Bielle sup (Autodesk Fusion 360 design; units mm, degrees)
Autodesk Fusion 360 part; units mm, degrees
sketch "Sketch1" plane through (0, 0, 0) normal (0, 0, 1) x (1, 0, 0) in component "Grande Bielle"
  line L0 (-178.5, 0) -> (178.5, 0) construction
  line L1 (-20, -20) -> (20, -20)
  line L2 (-32.5, 20) -> (-165, 7.5464)
  line L3 (20, -20) -> (165, -7.4425)
  line L4 (-20, -20) -> (-165, -7.4425)
  circle A0 centre (-178.5, 0) radius 3 construction
  line L5 (32.5, 20) -> (165, 7.5464)
  line L6 (0, 20) -> (0, -20) construction
  circle A1 centre (178.5, 0) radius 3 construction
  line L7 (32.5, 20) -> (32.5, 25)
  line L8 (32.5, 25) -> (-32.5, 25)
  line L9 (-32.5, 25) -> (-32.5, 20)
  line L10 (19.4422, 5.1) -> (-19.4422, -5.1) construction
  line L11 (-19.4422, 5.1) -> (19.4422, -5.1) construction
  arc A2 (-19.4422, 5.1) -> (-19.4422, -5.1) centre (0, 0) ccw
  arc A3 (19.4422, -5.1) -> (19.4422, 5.1) centre (0, 0) ccw
  line L12 (-32.5, 20) -> (32.5, 20) construction
  arc A4 (-14.2127, -5.1) -> (14.2127, -5.1) centre (0, 0) ccw
  arc A5 (14.2127, 5.1) -> (-14.2127, 5.1) centre (0, 0) ccw
  line L13 (19.4422, 5.1) -> (14.2127, 5.1)
  line L14 (-14.2127, 5.1) -> (-19.4422, 5.1)
  line L15 (-19.4422, -5.1) -> (-14.2127, -5.1)
  line L16 (14.2127, -5.1) -> (19.4422, -5.1)
  line L17 (-165, 7.5464) -> (-165, -7.4425)
  circle A6 centre (-155, 0) radius 2.1
  circle A7 centre (-145, 0) radius 2.1
  line L18 (165, 7.5464) -> (165, -7.4425)
  circle A8 centre (155, 0) radius 2.1
  circle A9 centre (145, 0) radius 2.1
  point P0 (0, 20)
  dimension "d1" = 357
  dimension "d2" = 6
  dimension "d3" = 6
  dimension "d8" = 20
  dimension "d9" = 65
  dimension "d10" = 20
  dimension "d13" = 5
  dimension "d63" = 40.2
  dimension "d64" = 10.2
  dimension "d65" = 20.1
  dimension "d272" = 40
  dimension "d274" = 15.1
  dimension "d275" = 15.1
  dimension "d297" = 165
  dimension "d298" = 4.2
  dimension "d299" = 10
  dimension "d300" = 4.2
  dimension "d301" = 10
  dimension "d302" = 165
  dimension "d303" = 4.2
  dimension "d304" = 4.2
  dimension "d305" = 10
  dimension "d306" = 10
  constraint horizontal L0
  constraint coincident L0.start A0.centre
  constraint coincident L0.end A1.centre
  constraint midpoint A2.centre L0
  constraint perpendicular L0 L6
  constraint midpoint L6.end L1
  constraint horizontal L1
  constraint coincident A2.centre A3.centre
  constraint vertical L7
  constraint horizontal L8
  constraint vertical L9
  constraint parallel L13 L15
  constraint horizontal L13
  constraint coincident L10.start A2
  constraint coincident L10 A2.centre
  constraint coincident L11 A2.centre
  constraint coincident P0 L6.start
  constraint coincident L5.start L7.start
  constraint coincident L6 A2.centre
  constraint perpendicular L6 L12
  constraint midpoint P0 L12
  constraint coincident A5.end L13
  constraint concentric A4 A5
  constraint coincident A4.end L15
  constraint collinear L13 L14
  constraint collinear L15 L16
  constraint vertical L17
  constraint coincident L0 A6.centre
  constraint coincident L0 A7.centre
  constraint perpendicular L0 L18
  constraint coincident L0 A8.centre
  constraint coincident L0 A9.centre
  measures "d1" distance of L0.start L0.end
  measures "d2" diameter of A0
  measures "d3" diameter of A1
  measures "d8" distance of A2.centre L6.end
  measures "d9" distance of L2.start L5.start
  measures "d10" vertical distance of A2.centre P0
  measures "d13" distance of L2.start L8.end
  measures "d63" diameter of A2
  measures "d64" distance of L11.start L10.end
  measures "d65" radius of A3
  measures "d272" distance of L1.end L1.start
  measures "d274" radius of A5
  measures "d275" radius of A4
  measures "d297" horizontal distance of L6.end L4.end
  measures "d298" diameter of A6
  measures "d299" distance of L17 A6.centre
  measures "d300" diameter of A7
  measures "d301" distance of A6.centre A7.centre
  measures "d302" distance of A2.centre L18
  measures "d303" diameter of A8
  measures "d304" diameter of A9
  measures "d305" distance of L18 A8.centre
  measures "d306" distance of A8.centre A9.centre
extrude "Extrude1" add sketch "Sketch1" along normal blind 10 makes body 1 in component "Grande Bielle"
sketch "Sketch6" plane through (0, 0, 10) normal (0, 0, 1) x (-1, 0, 0) in component "Fixation rotule"
  circle A0 centre (-145, 0) radius 2.1
  circle A1 centre (-155, 0) radius 2.1
  circle A2 centre (155, 0) radius 2.1
  line L0 (-19.4422, 5.1) -> (-14.2127, 5.1)
  arc A3 (14.2127, 5.1) -> (-14.2127, 5.1) centre (0, 0) ccw
  line L1 (14.2127, 5.1) -> (19.4422, 5.1)
  arc A4 (19.4422, -5.1) -> (19.4422, 5.1) centre (0, 0) ccw
  line L2 (19.4422, -5.1) -> (14.2127, -5.1)
  arc A5 (-14.2127, -5.1) -> (14.2127, -5.1) centre (0, 0) ccw
  line L3 (-14.2127, -5.1) -> (-19.4422, -5.1)
  arc A6 (-19.4422, 5.1) -> (-19.4422, -5.1) centre (0, 0) ccw
  circle A7 centre (145, 0) radius 2.1
  line L4 (-32.5, -20) -> (-32.5, -25)
  line L5 (-32.5, -25) -> (32.5, -25)
  line L6 (32.5, -25) -> (32.5, -20)
  line L7 (32.5, -20) -> (165, -7.5464)
  line L8 (165, -7.5464) -> (165, 7.4425)
  line L9 (165, 7.4425) -> (20, 20)
  line L10 (20, 20) -> (-20, 20)
  line L11 (-20, 20) -> (-165, 7.4425)
  line L12 (-165, 7.4425) -> (-165, -7.5464)
  line L13 (-165, -7.5464) -> (-32.5, -20)
  line L14 (169, -9.3299) -> (183.1865, -9.0359)
  circle A8 centre (155, 0) radius 2.1
  line L15 (167, -7.5091) -> (167, 7.4199)
  line L16 (169, -9.3299) -> (169, 9.2542)
  line L17 (165, -7.5464) -> (165, 7.4425) construction
  circle A9 centre (145, 0) radius 2.1
  line L18 (167, -7.5091) -> (169, -7.5091)
  line L19 (134, -12.6196) -> (169, -9.3299)
  line L20 (167, -7.5091) -> (134, -10.6107)
  line L21 (169, -0.0379) -> (183, -0.0379) construction
  circle A10 centre (145, 0) radius 2.1 construction
  circle A11 centre (155, 0) radius 2.1 construction
  circle A12 centre (183, -0.0379) radius 9
  circle A13 centre (155, 0) radius 2.1
  line L22 (165, -7.5464) -> (165, 7.4425)
  line L23 (167, 7.4199) -> (169, 7.4199)
  line L24 (169, 9.2542) -> (183.1865, 8.9602)
  line L25 (167, 7.4199) -> (134, 10.2778)
  circle A14 centre (145, 0) radius 2.1
  circle A15 centre (183, -0.0379) radius 3.1
  line L26 (169, 9.2542) -> (134, 12.2853)
  line L27 (134, 12.2853) -> (134, -12.6196)
  dimension "d432" = 4
  dimension "d433" = 35
  dimension "d434" = 2
  dimension "d435" = 2
  dimension "d436" = 2
  dimension "d437" = 6.2
  dimension "d438" = 18
  dimension "d439" = 28
  constraint vertical L16
  constraint parallel L16 L27
  constraint parallel L15 L17
  constraint coincident L25.end L27
  constraint parallel L25 L26
  constraint coincident L20.end L27
  constraint concentric A8 A11
  constraint concentric A10 A14
  constraint midpoint L21.start L16
  constraint perpendicular L16 L21
  constraint coincident L21.end A12.centre
  constraint concentric A12 A15
  constraint coincident L14.end A12
  constraint tangent L14 A12
  constraint coincident L24.end A12
  constraint tangent A12 L24
  constraint coincident L18.end L16
  constraint perpendicular L16 L18
  constraint coincident L23.end L16
  constraint perpendicular L16 L23
  measures "d432" distance of L16 L17
  measures "d433" distance of L16 L27
  measures "d434" distance of L15 L17
  measures "d435" distance of L19 L20
  measures "d436" distance of L25 L26
  measures "d437" diameter of A15
  measures "d438" diameter of A12
  measures "d439" horizontal distance of A2.centre L21.end
extrude "Extrude1'" add sketch "Sketch6" along normal mid plane 14 separate body contours L7 L8 L9 L22 L27 | L7 L8 L9 L15 L20 L22 L25 L27 | L16 L18 L19 L20 L27 | L16 L23 L25 L26 L27 | L15 L16 L18 L23 | L14 L16 A12 L24 | A12 makes body 2 in component "Fixation rotule"
extrude "Extrude2" cut sketch "Sketch6" along normal mid plane 11 contours L7 L8 L9 L22 L27 | L7 L8 L9 L15 L20 L22 L25 L27 bodies 2 in component "Fixation rotule"
extrude "Extrude3" cut sketch "Sketch6" along normal mid plane 9 contours L14 L16 A12 L24 | A12 bodies 2 in component "Fixation rotule"
fillet "Fillet1" radius 5 2 edges at (-169, 0.0379, 14.5) (-169, 0.0379, 5.5) on bodies 2 in component "Fixation rotule"
sketch "Sketch1 (2)" plane through (0.0705, -0.1, 10) normal (0, 0, 1) x (-1, 0, 0) in component "Axe centrale V2"
  circle A0 centre (-144.9295, -0.1) radius 2.1
  circle A1 centre (-154.9295, -0.1) radius 2.1
  circle A2 centre (155.0705, -0.1) radius 2.1
  line L0 (-19.3717, 5) -> (-14.1421, 5)
  arc A3 (14.2832, 5) -> (-14.1421, 5) centre (0.0705, -0.1) ccw
  line L1 (14.2832, 5) -> (19.5128, 5)
  arc A4 (19.5128, -5.2) -> (19.5128, 5) centre (0.0705, -0.1) ccw
  line L2 (19.5128, -5.2) -> (14.2832, -5.2)
  arc A5 (-14.1421, -5.2) -> (14.2832, -5.2) centre (0.0705, -0.1) ccw
  line L3 (-14.1421, -5.2) -> (-19.3717, -5.2)
  arc A6 (-19.3717, 5) -> (-19.3717, -5.2) centre (0.0705, -0.1) ccw
  circle A7 centre (145.0705, -0.1) radius 2.1
  line L4 (-32.4295, -20.1) -> (-32.4295, -25.1)
  line L5 (-32.4295, -25.1) -> (32.5705, -25.1)
  line L6 (32.5705, -25.1) -> (32.5705, -20.1)
  line L7 (32.5705, -20.1) -> (165.0705, -7.6464)
  line L8 (165.0705, -7.6464) -> (165.0705, 7.3425)
  line L9 (165.0705, 7.3425) -> (20.0705, 19.9)
  line L10 (20.0705, 19.9) -> (-19.9295, 19.9)
  line L11 (-19.9295, 19.9) -> (-164.9295, 7.3425)
  line L12 (-164.9295, 7.3425) -> (-164.9295, -7.6464)
  line L13 (-164.9295, -7.6464) -> (-32.4295, -20.1)
  line L14 (-14.1421, -5.2) -> (-19.3717, -5.2)
  arc A8 (-14.1421, -5.2) -> (14.2832, -5.2) centre (0.0705, -0.1) ccw
  line L15 (19.5128, -5.2) -> (14.2832, -5.2)
  arc A9 (19.5128, -5.2) -> (19.5128, 5) centre (0.0705, -0.1) ccw
  line L16 (14.2832, 5) -> (19.5128, 5)
  arc A10 (14.2832, 5) -> (-14.1421, 5) centre (0.0705, -0.1) ccw
  line L17 (-19.3717, 5) -> (-14.1421, 5)
  arc A11 (-19.3717, 5) -> (-19.3717, -5.2) centre (0.0705, -0.1) ccw
  circle A12 centre (0.0705, -0.1) radius 22
  dimension "d516" = 44
  constraint concentric A3 A12
  measures "d516" diameter of A12
extrude "Extrude1''" add sketch "Sketch1 (2)" against normal blind 5 separate body contours L0 A3 L1 A4 L2 A5 L3 A6 L14 A8 L15 A9 L16 A10 L17 A11 makes body 3 in component "Axe centrale V2"
extrude "Extrude2'" add sketch "Sketch1 (2)" along normal blind 3 contours L0 A3 L1 A4 L2 A5 L3 A6 L14 A8 L15 A9 L16 A10 L17 A11 | L10 A12 | L10 A12 bodies 3 in component "Axe centrale V2"
sketch "Sketch2" plane through (0, 0, 13) normal (0, 0, 1) x (-1, 0, 0) in component "Axe centrale V2"
  circle A0 centre (0, 0) radius 22
  circle A1 centre (0, 0) radius 11.1
  circle A2 centre (0, 0) radius 7.5
  dimension "d521" = 22.2
  dimension "d522" = 15
  constraint coincident A0.centre A1.centre
  constraint concentric A0 A2
  measures "d521" diameter of A1
  measures "d522" diameter of A2
extrude "Extrude3'" cut sketch "Sketch2" against normal through all contours A2 bodies 3 in component "Axe centrale V2"
extrude "Extrude4" cut sketch "Sketch2" against normal blind 7 contours A1 bodies 3 in component "Axe centrale V2"
sketch "Sketch1 (3)" plane through (0, 0, 0) normal (0, 0, 1) x (1, 0, 0) in component "Rolling v2"
  circle A0 centre (0, 0) radius 11
  circle A1 centre (0, 0) radius 4
  circle A2 centre (0, 0) radius 10
  circle A3 centre (0, 0) radius 5
  dimension "d1_1" = 22
  dimension "d2_1" = 8
  dimension "d5" = -1
  dimension "d6" = 1
  constraint coincident A0.centre A1.centre
  measures "d1_1" diameter of A0
  measures "d2_1" diameter of A1
extrude "Extrude2''" add sketch "Sketch1 (3)" along normal blind 7 separate body contours A0 makes body 4 in component "Rolling v2"
fillet "Fillet1'" radius 0.2 2 edges at (-10.2556, -3.9778, 7) (-9.3233, 3.6162, 7) on bodies 4 in component "Rolling v2"
fillet "Fillet1'" radius 0.2 2 edges at (-10.2556, -3.9778, 0) (-9.3233, 3.6162, 0) on bodies 4 in component "Rolling v2"
extrude "Extrude3''" add sketch "Sketch1 (3)" along normal blind 7 separate body contours A3 makes body 5 in component "Rolling v2"
fillet "Fillet2" radius 0.2 2 edges at (-4.6616, -1.8081, 7) (-3.7293, 1.4465, 7) on bodies 5 in component "Rolling v2"
fillet "Fillet2" radius 0.2 2 edges at (-4.6616, -1.8081, 0) (-3.7293, 1.4465, 0) on bodies 5 in component "Rolling v2"
extrude "Extrude4'" add sketch "Sketch1 (3)" along normal blind 7 separate body contours A2 makes body 6 in component "Rolling v2"
fillet "Fillet3" radius 0.2 2 edges at (-9.3233, -3.6162, 7) (-4.6616, 1.8081, 7) on bodies 6 in component "Rolling v2"
fillet "Fillet3" radius 0.2 2 edges at (-9.3233, -3.6162, 0) (-4.6616, 1.8081, 0) on bodies 6 in component "Rolling v2"
combine "Combine1" operation add target body 4 tool bodies 5 6 in component "Rolling v2"
sketch "Sketch1 (4)" plane through (0, 0, 0) normal (0, 0, 1) x (1, 0, 0) in component "Rolling v2 (1)"
  circle A0 centre (0, 0) radius 11
  circle A1 centre (0, 0) radius 4
  circle A2 centre (0, 0) radius 10
  circle A3 centre (0, 0) radius 5
  dimension "d1_2" = 22
  dimension "d2_2" = 8
  dimension "d5_1" = -1
  dimension "d6_1" = 1
  constraint coincident A0.centre A1.centre
  measures "d1_2" diameter of A0
  measures "d2_2" diameter of A1
extrude "Extrude2'''" add sketch "Sketch1 (4)" along normal blind 7 separate body contours A0 makes body 7 in component "Rolling v2 (1)"
fillet "Fillet1''" radius 0.2 2 edges at (-10.2556, -3.9778, 7) (-9.3233, 3.6162, 7) on bodies 7 in component "Rolling v2 (1)"
fillet "Fillet1''" radius 0.2 2 edges at (-10.2556, -3.9778, 0) (-9.3233, 3.6162, 0) on bodies 7 in component "Rolling v2 (1)"
extrude "Extrude3'''" add sketch "Sketch1 (4)" along normal blind 7 separate body contours A3 makes body 8 in component "Rolling v2 (1)"
fillet "Fillet2'" radius 0.2 2 edges at (-4.6616, -1.8081, 7) (-3.7293, 1.4465, 7) on bodies 8 in component "Rolling v2 (1)"
fillet "Fillet2'" radius 0.2 2 edges at (-4.6616, -1.8081, 0) (-3.7293, 1.4465, 0) on bodies 8 in component "Rolling v2 (1)"
extrude "Extrude4''" add sketch "Sketch1 (4)" along normal blind 7 separate body contours A2 makes body 9 in component "Rolling v2 (1)"
fillet "Fillet3'" radius 0.2 2 edges at (-9.3233, -3.6162, 7) (-4.6616, 1.8081, 7) on bodies 9 in component "Rolling v2 (1)"
fillet "Fillet3'" radius 0.2 2 edges at (-9.3233, -3.6162, 0) (-4.6616, 1.8081, 0) on bodies 9 in component "Rolling v2 (1)"
combine "Combine1'" operation add target body 7 tool bodies 8 9 in component "Rolling v2 (1)"
component "Grande Bielle" placed x (1, 0, 0) y (0, 1, 0) z (0, 0, 1) at (0, 0, 0)
component "Fixation rotule" placed x (1, 0, 0) y (0, 1, 0) z (0, 0, 1) at (0, 0, -5.5)
component "Fixation rotule" placed x (-1, 0, 0) y (0, -1, 0) z (0, 0, 1) at (0, 0, -4.5)
component "Axe centrale V2" placed x (1, 0, 0) y (0, -1, 0) z (0, 0, -1) at (0, 0, 10)
component "Rolling v2" placed x (1, 0, 0) y (0, -1, 0) z (0, 0, -1) at (0, 0, 4)
component "Axe centrale V2" placed x (1, 0, 0) y (0, 1, 0) z (0, 0, 1) at (0, 0, 0)
component "Rolling v2 (1)" placed x (1, 0, 0) y (0, 1, 0) z (0, 0, 1) at (0, 0, 6)
named bodies: "Axe centrale V2"
